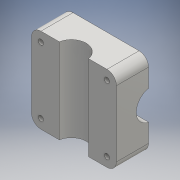
# Autodesk Inventor part: Middle
Saved by Autodesk Inventor 2016 (Build 200138000, 138)
## iProperties
Created: 2017-02-05
Part Number: Middle
Material: PC/ABS Plastic
Document SubType Name: Modeling
Designer: Liquid Metal Printer
Density: 0.357273 g/cm^3
Appearance: Smooth - White
Author: Liquid Metal Printer
Autodesk Inventor part; units mm, degrees
ref_plane "YZ Plane" through (0, 0, 0) normal (1, 0, 0) x (0, 1, 0)
ref_plane "XZ Plane" through (0, 0, 0) normal (0, 1, 0) x (-1, 0, 0)
ref_plane "XY Plane" through (0, 0, 0) normal (0, 0, 1) x (1, 0, 0)
sketch "Sketch1" plane through (0, 0, 0) normal (0, 1, 0) x (-1, 0, 0)
  line L0 (45, -5) -> (45, -14.75)
  line L1 (45, -14.75) -> (45, -30.25)
  line L2 (45, -30.25) -> (45, -40)
  arc A0 (40, -45) -> (45, -40) centre (40, -40) ccw
  circle A1 centre (40, -40) radius 1.375
  circle A2 centre (40, -5) radius 1.375
  arc A3 (45, -5) -> (40, 0) centre (40, -5) ccw
  line L3 (5, 0) -> (40, 0)
  circle A4 centre (5, -5) radius 1.375
  arc A5 (5, 0) -> (0, -5) centre (5, -5) ccw
  line L4 (0, -14.75) -> (0, -5)
  line L5 (0, -30.25) -> (0, -14.75)
  line L6 (0, -40) -> (0, -30.25)
  arc A6 (0, -40) -> (5, -45) centre (5, -40) ccw
  line L7 (40, -45) -> (5, -45)
  circle A7 centre (5, -40) radius 1.375
  point P0 (0, 0)
  point P1 (0, 0)
  constraints: 16 end point, 8 centre point, 8 point on circle
extrude "Extrusion1" add sketch "Sketch1" along normal blind 17
sketch "Sketch2" plane through (0, 0, -5) normal (1, 0, 0) x (0, 0, -1)
  line L0 (35, 0) -> (0, 0) projected
  line L1 (35, 0) -> (35, 17) projected
  line L2 (0, 17) -> (35, 17) projected
  line L3 (0, 0) -> (0, 17) projected
  line L4 (-5, 0) -> (-5, 17) projected
  line L5 (40, 0) -> (35, 0) projected
  line L6 (40, 0) -> (40, 17) projected
  line L7 (35, 17) -> (40, 17) projected
  line L8 (35, 0) -> (35, 17) projected
  line L9 (0, 0) -> (-5, 0) projected
  line L10 (0, 0) -> (0, 17) projected
  line L11 (-5, 17) -> (0, 17) projected
  line L12 (-5, 0) -> (-5, 17) projected
  line L13 (35, 17) -> (0, 17) projected
  line L14 (0, 0) -> (35, 0) projected
  line L15 (17.5, 17) -> (25.25, 17)
  line L16 (25.25, 17) -> (9.75, 17)
  line L17 (17.5, 17) -> (17.5, 10.5)
  arc A0 (9.75, 17) -> (25.25, 17) centre (17.5, 18.3702) ccw
  dimension "d8" = 7.75
  dimension "d9" = 15.5
  dimension "d10" = 6.5
  constraints: 6 end point, 3 point on circle, 2 point on line, 1 centre point, 1 midpoint, 1 perpendicular
  measures "d8" distance of L15.start L15.end
  measures "d9" distance of L15.end L16.end
  measures "d10" distance of L15.start L17.end
extrude "Extrusion2" cut sketch "Sketch2" against normal blind 45 contours A0 L17 L2 | L2 L17 A0
sketch "Sketch3" plane through (-40, 0, 0) normal (0, 0, 1) x (1, 0, 0)
  line L0 (35, 0) -> (0, 0) projected
  line L1 (35, 0) -> (35, 17) projected
  line L2 (0, 17) -> (35, 17) construction
  line L3 (0, 0) -> (0, 17) projected
  line L4 (17.5, 0) -> (9.75, 0)
  line L5 (9.75, 0) -> (25.25, 0)
  line L6 (17.5, 0) -> (17.5, 6.5)
  arc A0 (25.25, 0) -> (9.75, 0) centre (17.5, -1.3702) ccw
  line L7 (35, 0) -> (0, 0) projected
  point P0 (40, 0)
  point P1 (17.5, 0)
  dimension "d13" = 7.75
  dimension "d14" = 15.5
  dimension "d15" = 6.5
  constraints: 6 end point, 3 point on circle, 1 centre point, 1 midpoint, 1 perpendicular
  measures "d13" distance of L4.start L4.end
  measures "d14" distance of L4.end L5.end
  measures "d15" distance of L4.start L6.end
extrude "Extrusion3" cut sketch "Sketch3" against normal blind 45
body "Solid1"
